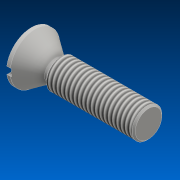
# Autodesk Inventor part: parafuso escariado M3,5
Saved by Autodesk Inventor 2016 (Build 200138000, 138)
## iProperties
Created: 2018-11-29
Part Number: parafuso escariado M3,5
Material: Generic
Document SubType Name: Modeling
Designer: lesly
Density: 1 g/cm^3
Appearance: Default
Author: lesly
Autodesk Inventor part; units mm, degrees
ref_plane "YZ Plane" through (0, 0, 0) normal (1, 0, 0) x (0, 1, 0)
ref_plane "XZ Plane" through (0, 0, 0) normal (0, 1, 0) x (-1, 0, 0)
ref_plane "XY Plane" through (0, 0, 0) normal (0, 0, 1) x (1, 0, 0)
sketch "Sketch2" plane through (0, 0, 0) normal (1, 0, 0) x (0, 1, 0)
  circle A0 centre (0, 0) radius 1.75
  constraints: 1 centre point, 1 coincident
extrude "Extrusion1" add sketch "Sketch2" along normal mid plane 10.2
chamfer "Chamfer1" distance 0.2 angle 45 1 edges at (5.1, -1.75, 0) measured on face at (5.1, -0.5165, 0.5026)
sketch "Sketch3" plane through (-5.1, 0, 0) normal (-1, 0, 0) x (0, 0, 1)
  circle A0 centre (0, 0) radius 1.75
  dimension "d27" = 3.5
  constraints: 1 centre point, 1 coincident
  measures "d27" diameter of A0
extrude "Extrusion2" add sketch "Sketch3" along normal blind 0.32
chamfer "Chamfer2" distance 0.32 angle 45 1 edges at (-5.42, 0, -1.75) measured on face at (-5.42, 0.5026, -0.5165)
sketch "Sketch4" plane through (-5.42, 0, 0) normal (-1, 0, 0) x (0, 0, 1)
  circle A0 centre (0, 0) radius 1.25
  dimension "d33" = 2.5
  constraints: 1 centre point, 1 coincident
  measures "d33" diameter of A0
extrude "Extrusion3" add sketch "Sketch4" along normal blind 0.41
sketch "Sketch5" plane through (0, 0, 0) normal (0, 1, 0) x (-1, 0, 0)
  line L0 (5.83, 0) -> (5.83, -1.25)
  line L1 (8.63, -2.91) -> (8.21, -2.91)
  line L2 (8.21, -2.91) -> (5.83, -1.25)
  line L3 (8.63, -2.91) -> (8.63, 0)
  line L4 (5.83, -1.25) -> (5.83, 0)
  line L5 (8.63, 0) -> (5.83, 0)
  point P0 (0, 0)
  dimension "d40" = 0.42
  constraints: 12 end point, 2 vertical, 1 collinear, 1 horizontal, 1 perpendicular
  measures "d40" distance of L1.start L1.end
revolve "Revolution1" add sketch "Sketch5" angle 360 about axis through (-8.63, 0, 0) along (1, 0, 0)
sketch "Sketch6" plane through (-8.63, 0, 0) normal (-1, 0, 0) x (0, 0, 1)
  circle A0 centre (0, 0) radius 2.91 projected
  line L0 (0.425, 2.91) -> (0.425, -2.91)
  line L1 (-0.425, 2.91) -> (-0.425, -2.91)
  line L2 (-0.425, 2.91) -> (0.425, 2.91)
  line L3 (-0.425, -2.91) -> (0.425, -2.91)
  line L4 (-0.425, 2.91) -> (0.425, 2.91)
  line L5 (0.425, 2.91) -> (0.425, -2.91)
  line L6 (0.425, -2.91) -> (-0.425, -2.91)
  line L7 (-0.425, -2.91) -> (-0.425, 2.91)
  constraints: 16 end point, 3 horizontal, 2 parallel, 1 perpendicular
extrude "Extrusion4" cut sketch "Sketch6" against normal blind 0.5 contours L0 A0 L1 | A0 L2 L0 | L0 L3 A0 | A0 L1 L2 | L3 L1 A0
thread "Thread1" size "M4x0.5" class "6g" standard "ANSI Metric M Profile" full length
body "Solid1"
